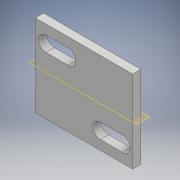
# Autodesk Inventor part: riser1.7mm
Saved by Autodesk Inventor 2017 (Build 210142000, 142)
## iProperties
Created: 2018-12-03
Part Number: riser1.7mm
Material: Generic
Document SubType Name: Modeling
Designer: Eric the Great
Density: 1 g/cm^3
Appearance: Default
Author: Eric the Great
Autodesk Inventor part; units mm, degrees
ref_plane "YZ Plane" through (0, 0, 0) normal (1, 0, 0) x (0, 1, 0)
ref_plane "XZ Plane" through (0, 0, 0) normal (0, 1, 0) x (-1, 0, 0)
ref_plane "XY Plane" through (0, 0, 0) normal (0, 0, 1) x (1, 0, 0)
sketch "Sketch1" plane through (0, 0, 0) normal (0, 1, 0) x (-1, 0, 0)
  line L0 (-13, 11) -> (13, 11)
  line L1 (13, 11) -> (13, -11)
  line L2 (13, -11) -> (-13, -11)
  line L3 (-13, -11) -> (-13, 11)
  line L4 (-13, 11) -> (13, -11) construction
  line L5 (13, 11) -> (-13, -11) construction
  line L6 (-4.3445, -6.4484) -> (-10.3445, -6.4484) construction
  line L7 (-4.3445, -4.4484) -> (-10.3445, -4.4484)
  line L8 (-10.3445, -8.4484) -> (-4.3445, -8.4484)
  arc A0 (-4.3445, -8.4484) -> (-4.3445, -4.4484) centre (-4.3445, -6.4484) ccw
  arc A1 (-10.3445, -4.4484) -> (-10.3445, -8.4484) centre (-10.3445, -6.4484) ccw
  line L9 (0, 0) -> (1.6306, 0)
  line L10 (10.1555, 6.4484) -> (4.1555, 6.4484) construction
  line L11 (10.1555, 8.4484) -> (4.1555, 8.4484)
  line L12 (4.1555, 4.4484) -> (10.1555, 4.4484)
  arc A2 (10.1555, 4.4484) -> (10.1555, 8.4484) centre (10.1555, 6.4484) ccw
  arc A3 (4.1555, 8.4484) -> (4.1555, 4.4484) centre (4.1555, 6.4484) ccw
  line L13 (0, 0) -> (1.2871, 0)
  point P0 (-7.3445, -6.4484)
  point P1 (7.1555, 6.4484)
  dimension "d0" = 26
  dimension "d1" = 22
  dimension "d5" = 6
  dimension "d6" = 4
  dimension "d16" = 6
  dimension "d17" = 4
  dimension "d18" = 14.5
  constraints: 32 end point, 8 point on circle, 8 tangent, 4 centre point, 4 horizontal, 4 midpoint, 4 parallel, 1 perpendicular, 1 point on line, 1 other
  measures "d0" distance of L1.end L2.end
  measures "d1" distance of L0.end L1.end
  measures "d5" distance of L6.start L6.end
  measures "d6" distance between parallel lines of L8 L7
  measures "d16" distance of L10.start L10.end
  measures "d17" distance between parallel lines of L12 L11
  measures "d18" horizontal distance of point (-7.344, -6.448) point (7.156, 6.448)
extrude "Extrusion1" add sketch "Sketch1" along normal blind 2.2
ref_plane "Work Plane1" through (-13, 0, 0) normal (0, 0, 1) x (1, 0, 0)
body "Solid1"
